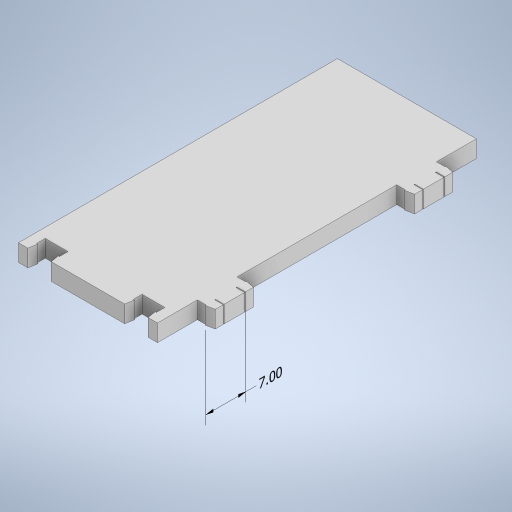
# Autodesk Inventor part: 左右
Saved by Autodesk Inventor 2024 (Build 280153000, 153)
## iProperties
Created: 2024-03-31
Part Number: 左右
Material: 一般
Document SubType Name: Modeling
Designer: USER
Density: 1 g/cm^3
Appearance: 預設
Author: USER
Autodesk Inventor part; units mm, degrees
ref_plane "YZ Plane" through (0, 0, 0) normal (1, 0, 0) x (0, 1, 0)
ref_plane "XZ Plane" through (0, 0, 0) normal (0, 1, 0) x (-1, 0, 0)
ref_plane "XY Plane" through (0, 0, 0) normal (0, 0, 1) x (1, 0, 0)
sketch "草圖1" plane through (0, 0, 0) normal (0, 1, 0) x (-1, 0, 0)
  line L0 (0, 0) -> (24.4, 0)
  line L1 (24.4, 0) -> (24.4, -56)
  line L2 (24.4, -56) -> (0, -56)
  line L3 (0, -56) -> (0, 0)
  line L4 (5.7, 0) -> (1.7, 0)
  line L5 (22.6499, 0) -> (18.7501, 0)
  line L6 (18.7, -2.9996) -> (22.7, -2.9996)
  line L7 (22.7, -2.9996) -> (22.7, -1.4996)
  line L8 (22.7, -1.4996) -> (22.5, -1.4996)
  line L9 (22.6499, 0) -> (22.7499, 0)
  line L10 (22.7499, 0) -> (22.5, -1.4996)
  line L11 (20.7, 0) -> (20.7, -2.9996)
  line L12 (18.7, -2.9996) -> (18.7, -1.4996)
  line L13 (18.7, -1.4996) -> (18.9, -1.4996)
  line L14 (18.6501, 0) -> (18.9, -1.4996)
  line L15 (12.2, 0) -> (12.2, -56)
  line L16 (5.7, -2.9996) -> (1.7, -2.9996)
  line L17 (1.7, -2.9996) -> (1.7, -1.4996)
  line L18 (1.7, -1.4996) -> (1.9, -1.4996)
  line L19 (1.6501, 0) -> (1.9, -1.4996)
  line L20 (5.7, -2.9996) -> (5.7, -1.4996)
  line L21 (5.7, -1.4996) -> (5.5, -1.4996)
  line L22 (5.7499, 0) -> (5.5, -1.4996)
  line L23 (0, -7) -> (-1.5, -7)
  line L24 (-1.5, -7) -> (-1.5, -6.85)
  line L25 (-3, -7.15) -> (-1.5, -6.85)
  line L26 (-3, -7.15) -> (-3, -8.55)
  line L27 (-3, -8.55) -> (-1.5, -8.55)
  line L28 (-1.5, -8.55) -> (-1.5, -8.7)
  line L29 (-1.5, -8.7) -> (-3, -8.7)
  line L30 (-3, -8.7) -> (-3, -10.5)
  line L31 (-3, -10.5) -> (0, -10.5)
  line L32 (0, -14) -> (-1.5, -14)
  line L33 (-1.5, -14) -> (-1.5, -14.15)
  line L34 (-3, -13.85) -> (-1.5, -14.15)
  line L35 (-3, -13.85) -> (-3, -12.45)
  line L36 (-3, -12.45) -> (-1.5, -12.45)
  line L37 (-1.5, -12.45) -> (-1.5, -12.3)
  line L38 (-1.5, -12.3) -> (-3, -12.3)
  line L39 (-3, -12.3) -> (-3, -10.5)
  line L40 (24.4, -28) -> (0, -28)
  line L41 (0, -49) -> (-1.5, -49)
  line L42 (-1.5, -49) -> (-1.5, -49.15)
  line L43 (-3, -48.85) -> (-1.5, -49.15)
  line L44 (-3, -48.85) -> (-3, -47.45)
  line L45 (-3, -47.45) -> (-1.5, -47.45)
  line L46 (-1.5, -47.45) -> (-1.5, -47.3)
  line L47 (-1.5, -47.3) -> (-3, -47.3)
  line L48 (-3, -47.3) -> (-3, -45.5)
  line L49 (-3, -45.5) -> (0, -45.5)
  line L50 (0, -42) -> (-1.5, -42)
  line L51 (-1.5, -42) -> (-1.5, -41.85)
  line L52 (-1.5, -43.55) -> (-1.5, -43.7)
  line L53 (-3, -42.15) -> (-3, -43.55)
  line L54 (-3, -43.55) -> (-1.5, -43.55)
  line L55 (-1.5, -43.7) -> (-3, -43.7)
  line L56 (-3, -43.7) -> (-3, -45.5)
  line L57 (-3, -42.15) -> (-1.5, -41.85)
  point P0 (0, -14)
  point P1 (0, -42)
  point P2 (18.6501, 0)
  point P3 (5.7499, 0)
  point P4 (1.6501, 0)
  dimension "d0" = 56
  dimension "d1" = 24.4
  dimension "d5" = 3
  dimension "d6" = 4
  dimension "d7" = 3.7
  dimension "d8" = 1.5
  dimension "d9" = 0.2
  dimension "d10" = 0.1
  dimension "d11" = 9.462
  dimension "d12" = 1.7
  dimension "d14" = 0.15
  dimension "d17" = 1.4
  dimension "d18" = 0.15
  dimension "d19" = 1.8
  dimension "d20" = 7
  dimension "d21" = 78.69
  dimension "d22" = 25.9
  dimension "d23" = 25.9
  dimension "d24" = 27.4
  dimension "d25" = 27.4
  dimension "d26" = 18.7
  dimension "d27" = 22.7
  dimension "d31" = 0.15
  constraints: 116 end point, 37 symmetric about line, 6 midpoint, 6 perpendicular, 4 horizontal, 4 parallel, 3 point on line, 3 vertical, 2 horizontal alignment
  measures "d0" distance of L2.end L0.start
  measures "d1" distance of L1.end L2.end
  measures "d5" distance of L5.end L6.start
  measures "d6" distance of L6.start L6.end
  measures "d7" distance of L0.end L11.start
  measures "d8" distance of L6.end L7.end
  measures "d9" distance of L7.end L8.end
  measures "d10" distance of L5.start L9.end
  measures "d11" angle of L10 L1
  measures "d12" distance between parallel lines of L7 L1
  measures "d14" distance of L23.end L24.end
  measures "d17" distance of L25.start L26.end
  measures "d18" distance of L27.end L28.end
  measures "d19" distance of L29.end L30.end
  measures "d20" distance of L23.start L0.start
  measures "d21" angle of L25 L1
  measures "d22" distance between parallel lines of L24 L1
  measures "d23" distance between parallel lines of L28 L1
  measures "d24" distance between parallel lines of L26 L1
  measures "d25" distance between parallel lines of L30 L1
  measures "d26" distance from line of L4.start L1
  measures "d27" distance from line of L4.end L1
  measures "d31" vertical distance of L25.start L23.end
extrude "擠出1" add sketch "草圖1" along normal blind 3 contours L0 L19 L18 L17 L16 L20 L21 L22 L15 L40 L3 | L3 L31 L30 L29 L28 L27 L26 L25 L24 L23 | L3 L32 L33 L34 L35 L36 L37 L38 L39 L31 | L40 L15 L2 L3 | L0 L14 L13 L12 L6 L7 L8 L10 L1 L40 L15 | L3 L49 L56 L55 L52 L54 L53 L57 L51 L50 | L40 L1 L2 L15 | L3 L41 L42 L43 L44 L45 L46 L47 L48 L49
